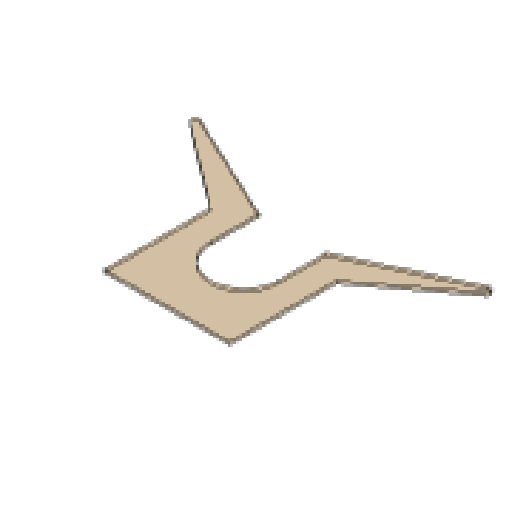
# Autodesk Inventor part: ConePlatform
Saved by Autodesk Inventor 2023 (Build 270158000, 158)
## iProperties
Created: 2022-11-09
Part Number: ConePlatform
Material: Polycarbonate, Smoke
Document SubType Name: Modeling
Designer: deli
Density: 1.2 g/cm^3
Appearance: Polycarbonate - Smoked
Author: deli
Autodesk Inventor part; units mm, degrees
ref_plane "YZ Plane" through (0, 0, 0) normal (1, 0, 0) x (0, 1, 0)
ref_plane "XZ Plane" through (0, 0, 0) normal (0, 1, 0) x (-1, 0, 0)
ref_plane "XY Plane" through (0, 0, 0) normal (0, 0, 1) x (1, 0, 0)
sketch "Sketch1" plane through (0, 0, 0) normal (0, 1, 0) x (-1, 0, 0)
  arc A0 (-9.5094, -8.2707) -> (-79.5094, -8.2707) centre (-44.5094, -8.2707) ccw
  line L0 (20.4906, 71.7293) -> (-109.5094, 71.7293)
  line L1 (-109.5094, 71.7293) -> (-109.5094, -38.2707)
  line L2 (20.4906, -38.2707) -> (20.4906, 71.7293)
  line L3 (-9.5094, -58.2707) -> (-9.5094, -8.2707)
  line L4 (-79.5094, -58.2707) -> (-79.5094, -8.2707)
  circle A1 centre (-44.5094, -8.2707) radius 80 construction
  line L5 (-79.5094, -58.2707) -> (-193.8106, -111.892)
  arc A2 (-197.921, -105.0793) -> (-193.8106, -111.892) centre (-195.5094, -108.2707) ccw
  line L6 (-109.5094, -38.2707) -> (-197.921, -105.0793)
  line L7 (-9.5094, -58.2707) -> (104.7917, -111.892)
  line L8 (20.4906, -38.2707) -> (108.9021, -105.0793)
  arc A3 (104.7917, -111.892) -> (108.9021, -105.0793) centre (106.4906, -108.2707) ccw
  point P0 (0, 0)
  dimension "d0" = 130
  dimension "d1" = 110
  dimension "d2" = 70
  dimension "d3" = 160
  dimension "d4" = 8
  dimension "d5" = 90
  dimension "d7" = 100
  dimension "d8" = 50
  dimension "d12" = 65
  constraints: 18 end point, 7 tangent, 6 point on circle, 4 centre point, 4 equal length, 2 parallel, 1 coincident, 1 equal radius, 1 horizontal, 1 perpendicular, 1 vertical
  measures "d0" distance of L0.start L0.end
  measures "d1" distance of L0.end L1.end
  measures "d2" diameter of A0
  measures "d3" diameter of A1
  measures "d4" diameter of A2
  measures "d7" vertical distance of A0.centre A2.centre
  measures "d8" distance of L4.start L4.end
  measures "d12" distance from line of L2 A0.centre
extrude "Extrusion1" add sketch "Sketch1" along normal blind 3.175
equation "\"d12\" = 0.5 * d0"
body "Solid1"
